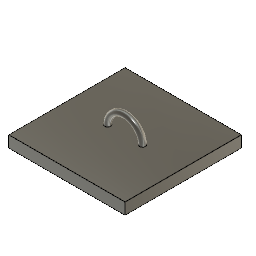
Tampa v2 (Autodesk Fusion 360 design; units mm, degrees)
Autodesk Fusion 360 part; units mm, degrees
sketch "Sketch1" plane through (0, 0, 0) normal (0, 0, 1) x (1, 0, 0)
  line L0 (50, -50) -> (-50, -50)
  line L1 (-50, -50) -> (-50, 50)
  line L2 (-50, 50) -> (50, 50)
  line L3 (50, 50) -> (50, -50)
  line L4 (50, -50) -> (-50, 50) construction
  line L5 (-50, -50) -> (50, 50) construction
  dimension "d1" = 100
  dimension "d2" = 100
  constraint horizontal L0
  constraint perpendicular L0 L1
  constraint parallel L0 L2
  constraint parallel L1 L3
  constraint coincident L4 origin
  constraint coincident L5 origin
  measures "d1" distance of L1.end L2.end
  measures "d2" distance of L0.end L1.end
extrude "Extrude1" add sketch "Sketch1" along normal blind 10
sketch "Sketch2" plane through (0, 50, 0) normal (0, 1, 0) x (-1, 0, 0)
  line L0 (-50, 0) -> (50, 0)
  line L1 (50, 0) -> (50, 10)
  line L2 (50, 10) -> (-50, 10)
  line L3 (-50, 10) -> (-50, 0)
  line L4 (-50, 0) -> (-40, 0)
  line L5 (-40, 0) -> (-40, 5)
  line L6 (-40, 5) -> (-30, 5)
  line L7 (-30, 5) -> (-30, 0)
  line L8 (-30, 0) -> (-40, 0)
  line L9 (50, 0) -> (40, 0)
  line L10 (40, 0) -> (40, 5)
  line L11 (40, 5) -> (30, 5)
  line L12 (30, 5) -> (30, 0)
  line L13 (30, 0) -> (40, 0)
  dimension "d14" = 10
  dimension "d15" = 5
  dimension "d16" = 10
  dimension "d17" = 5
  dimension "d18" = 10
  constraint coincident L0.start L3.end
  constraint perpendicular L3 L4
  constraint perpendicular L0 L5
  constraint perpendicular L5 L6
  constraint coincident L0 L7.end
  constraint perpendicular L0 L7
  constraint coincident L0.end L1.start
  constraint coincident L0 L9.end
  constraint perpendicular L1 L9
  constraint perpendicular L9 L10
  constraint perpendicular L10 L11
  constraint coincident L0 L12.end
  constraint perpendicular L0 L12
  measures "d14" distance of L0.start L4.end
  measures "d15" distance of L4.end L5.end
  measures "d16" distance of L5.end L6.end
  measures "d17" distance of L9.end L10.end
  measures "d18" distance of L10.end L11.end
extrude "Extrude3" add sketch "Sketch2" along normal blind 5 contours L0 L5 L6 L7 L8 | L0 L10 L11 L12 L13
sketch "Sketch3" plane through (40, 0, 0) normal (1, 0, 0) x (0, 1, 0)
  line L0 (50, 5) -> (50, 0)
  line L1 (50, 0) -> (55, 0)
  line L2 (55, 0) -> (55, 5)
  line L3 (55, 5) -> (50, 5)
  circle A0 centre (52.5, 2.5) radius 2
extrude "Extrude4" cut sketch "Sketch3" against normal blind 145 contours A0
sketch "Sketch4" plane through (0, 0, 0) normal (0, 1, 0) x (1, 0, 0)
  arc A0 (-15, -10) -> (15, -10) centre (0, -10) ccw
pipe "Pipe1" add diameter 5 wall 2 path "Sketch4" along A0
